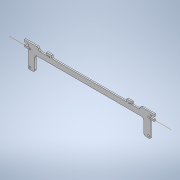
# Autodesk Inventor part: rod_4
Saved by Autodesk Inventor 2022 (Build 260153000, 153)
## iProperties
Created: 2023-04-07
Part Number: rod_4
Material: 一般
Document SubType Name: Modeling
Designer: may9c
Density: 79.16 g/cm^3
Appearance: 預設
Mass: 822.393 g
Surface Area: 88.4 cm^2
Volume: 10.389 cm^3
Author: may9c
Autodesk Inventor part; units mm, degrees
ref_plane "YZ Plane" through (0, 0, 0) normal (1, 0, 0) x (0, 1, 0)
ref_plane "XY Plane" through (0, 0, 0) normal (0, 0, 1) x (1, 0, 0)
sketch "草圖1" plane through (0, 0, 0) normal (0, 0, 1) x (1, 0, 0)
  line L0 (0, 6) -> (0, -6)
  line L1 (0, -6) -> (-139, -6)
  line L2 (-139, -6) -> (-139, 6)
  line L3 (-148, 2) -> (-139, 2)
  line L4 (-139, 2) -> (-139, -2)
  line L5 (-139, -2) -> (-148, -2)
  line L6 (-148, -2) -> (-148, 2)
  line L7 (-207.2, 0) -> (207.2, 0) projected
  line L8 (0, -9.6) -> (0, 15.6) projected
  line L9 (0, -6) -> (139, -6)
  line L10 (139, -6) -> (139, 6)
  line L11 (148, 2) -> (139, 2)
  line L12 (139, -2) -> (148, -2)
  line L13 (148, -2) -> (148, 2)
  line L14 (-148, -2) -> (-139, -2)
  line L15 (-139, -2) -> (-139, -6)
  line L16 (139, -6) -> (139, -2)
  line L17 (139, -2) -> (148, -2)
  line L18 (148, -2) -> (148, 2)
  line L19 (148, 2) -> (139, 2)
  line L20 (139, 2) -> (139, 6)
  line L21 (-139, 6) -> (-139, 2)
  line L22 (-139, 2) -> (-148, 2)
  line L23 (-148, 2) -> (-148, -2)
  line L24 (-97.5, 7) -> (-97.5, 12)
  line L25 (-97.5, 12) -> (-87.5, 12)
  line L26 (-90, 7) -> (-97.5, 7)
  line L27 (-90, 7) -> (-90, 5)
  line L28 (-90, 5) -> (-91, 5)
  line L29 (-91, 5) -> (-91, 6)
  line L30 (97.5, 7) -> (97.5, 12)
  line L31 (97.5, 12) -> (87.5, 12)
  line L32 (90, 7) -> (97.5, 7)
  line L33 (90, 7) -> (90, 5)
  line L34 (90, 5) -> (91, 5)
  line L35 (91, 5) -> (91, 6)
  line L36 (-139, 6) -> (-91, 6)
  line L37 (-85.5, 6) -> (85.5, 6)
  line L38 (91, 6) -> (139, 6)
  line L39 (-87.5, 12) -> (-85.5, 12)
  line L40 (-85.5, 12) -> (-85.5, 6)
  line L41 (87.5, 12) -> (85.5, 12)
  line L42 (85.5, 12) -> (85.5, 6)
  point P0 (0, 0)
  point P1 (-139, 2)
  dimension "d2" = 4
  dimension "d13" = 2
  dimension "d14" = 2
  dimension "d17" = 12
  constraints: 82 end point, 13 symmetric about line, 9 horizontal, 3 parallel, 3 perpendicular, 2 point on line, 1 collinear, 1 other
  measures "d2" distance between parallel lines of L5 L3
  measures "d13" distance of L25.end L39.end
  measures "d14" distance of L31.end L41.end
  measures "d17" distance between parallel lines of L1 L36
extrude "擠出1" add sketch "草圖1" along normal blind 3
ref_plane "工作平面1" through (0, 0, 1.5) normal (0, 0, 1) x (1, 0, 0)
sketch "草圖3" plane through (0, 0, 3) normal (0, 0, 1) x (1, 0, 0)
  line L0 (-148, 12.5) -> (-139, 12.5)
  line L1 (-139, 12.5) -> (-139, 7.5)
  line L2 (-139, 7.5) -> (-148, 7.5)
  line L3 (-148, 7.5) -> (-148, 12.5)
  line L4 (-139, 12.5) -> (-119, 12.5)
  arc A0 (-119, 6) -> (-115.75, 9.25) centre (-119, 9.25) ccw construction
  arc A1 (-115.75, 9.25) -> (-112.5, 6) centre (-112.5, 9.25) ccw
  line L5 (-91, 6) -> (-139, 6) projected
  line L6 (-148, 2) -> (-148, -2) projected
  line L7 (-139, 2) -> (-148, 2) projected
  line L8 (-139, 7.5) -> (-139, 6)
  arc A2 (-119, 12.5) -> (-119, 6) centre (-119, 9.25) ccw construction
  arc A3 (-115.75, 9.25) -> (-119, 12.5) centre (-119, 9.25) ccw
  arc A4 (-112.5, 6) -> (-115.75, 9.25) centre (-112.5, 9.25) ccw construction
  point P0 (0, 0)
  dimension "d20" = 20
  dimension "d21" = 5.5
  dimension "d22" = 5
  constraints: 12 end point, 10 point on circle, 6 tangent, 5 centre point, 3 parallel, 2 horizontal, 2 point on line, 1 collinear, 1 equal radius, 1 perpendicular, 1 vertical
  measures "d20" distance of L0.end L4.end
  measures "d21" distance between parallel lines of L7 L2
  measures "d22" distance between parallel lines of L2 L0
extrude "擠出2" add sketch "草圖3" against normal up to surface (3 mm away)
mirror "鏡射2" about plane through (0, 0, 0) normal (1, 0, 0) of "擠出2"
sketch "草圖4" plane through (0, 0, 3) normal (0, 0, 1) x (1, 0, 0)
  circle A0 centre (-135.5, 0) radius 6.5
  line L0 (207.2, 0) -> (-207.2, 0) projected
  line L1 (-139, 2) -> (-148, 2) projected
  line L2 (-142, 2) -> (-142, -2)
  line L3 (-148, -2) -> (-139, -2) projected
  line L4 (-148, 2) -> (-148, -2) projected
  line L5 (-139, 2) -> (-139, 7.5) projected
  circle A1 centre (-135.5, 0) radius 2.05
  point P0 (0, 0)
  dimension "d25" = 13
  dimension "d26" = 6
  dimension "d27" = 4.1
  constraints: 3 point on line, 2 centre point, 2 end point, 1 tangent, 1 vertical
  measures "d25" diameter of A0
  measures "d26" distance between parallel lines of L4 L2
  measures "d27" diameter of A1
extrude "擠出3" cut sketch "草圖4" against normal up to surface (3 mm away) contours A1 L0 | L0 A1
sketch "草圖5" plane through (0, 0, 3) normal (0, 0, 1) x (1, 0, 0)
  line L0 (-139, -6) -> (139, -6) projected
  line L1 (-139, -6) -> (-139, -39)
  line L2 (-137, -41) -> (-129, -41)
  line L3 (-124, -36) -> (-124, -11)
  arc A0 (-119, -6) -> (-124, -11) centre (-119, -11) ccw
  circle A1 centre (-135.5, 0) radius 2.05 projected
  circle A2 centre (-135.5, -36) radius 2.05
  arc A3 (-129, -41) -> (-124, -36) centre (-129, -36) ccw
  arc A4 (-139, -39) -> (-137, -41) centre (-137, -39) ccw
  point P0 (0, 0)
  point P1 (-139, -41)
  point P2 (-124, -41)
  dimension "d30" = 35
  dimension "d31" = 15
  dimension "d32" = 10
  dimension "d33" = 5
  dimension "d35" = 5
  dimension "d36" = 2
  constraints: 6 end point, 6 point on circle, 6 tangent, 5 point on line, 4 centre point, 2 perpendicular, 1 equal radius, 1 vertical, 1 vertical alignment
  measures "d30" distance of L0.start point (-139, -41)
  measures "d31" distance of point (-139, -41) point (-124, -41)
  measures "d32" diameter of A0
  measures "d33" distance from line of L2 A2.centre
  measures "d35" radius of A3
  measures "d36" radius of A4
extrude "擠出4" add sketch "草圖5" against normal up to surface (3 mm away) contours L0 A0 L3 A3 L2 A4 L1
mirror "鏡射3" about plane through (0, 0, 0) normal (1, 0, 0) of "擠出4", "擠出3"
